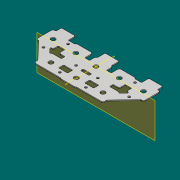
# Autodesk Inventor part: Part2
Saved by Autodesk Inventor 2018 (Build 220112000, 112)
## iProperties
Created: 2021-10-17
Part Number: Part2
Material: アルミニウム 6061
Document SubType Name: Modeling
Designer: gisen
Density: 2.7 g/cm^3
Appearance: アルミニウム - フラット
Author: gisen
Autodesk Inventor part; units mm, degrees
ref_plane "YZ Plane" through (0, 0, 0) normal (1, 0, 0) x (0, 1, 0)
ref_plane "XY Plane" through (0, 0, 0) normal (0, 0, 1) x (1, 0, 0)
ref_plane "作業平面1" through (0, -39.175, 8.3) normal (0, 0, -1) x (-1, 0, 0)
sketch "スケッチ1" plane through (0, -39.175, 8.3) normal (0, 0, -1) x (-1, 0, 0)
  arc A0 (-5.35, 6.375) -> (-6.35, 5.375) centre (-5.35, 5.375) ccw construction
  arc A1 (6.35, 5.375) -> (5.35, 6.375) centre (5.35, 5.375) ccw construction
  arc A2 (-32.9, 5.375) -> (-33.9, 6.375) centre (-33.9, 5.375) ccw construction
  arc A3 (-44.6, 6.375) -> (-45.6, 5.375) centre (-44.6, 5.375) ccw construction
  arc A4 (33.9, 6.375) -> (32.9, 5.375) centre (33.9, 5.375) ccw construction
  arc A5 (45.6, 5.375) -> (44.6, 6.375) centre (44.6, 5.375) ccw construction
  arc A6 (48.3, -0.325) -> (46.5, 1.475) centre (46.5, -0.325) ccw construction
  arc A7 (46.5, -13.925) -> (48.3, -12.125) centre (46.5, -12.125) ccw construction
  arc A8 (-46.5, 1.475) -> (-48.3, -0.325) centre (-46.5, -0.325) ccw construction
  arc A9 (-48.3, -12.125) -> (-46.5, -13.925) centre (-46.5, -12.125) ccw construction
  arc A10 (-17.5, -33.025) -> (-15.7, -31.225) centre (-17.5, -31.225) ccw construction
  arc A11 (15.7, -31.225) -> (17.5, -33.025) centre (17.5, -31.225) ccw construction
  arc A12 (31.1, -19.425) -> (29.3, -17.625) centre (29.3, -19.425) ccw construction
  arc A13 (-5.9, -0.585) -> (-7.7, -2.385) centre (-5.9, -2.385) ccw construction
  arc A14 (7.7, -2.385) -> (5.9, -0.585) centre (5.9, -2.385) ccw construction
  arc A15 (13.6, 0.875) -> (12.2994, 0.3193) centre (13.6, -0.925) ccw construction
  arc A16 (27.2, -0.925) -> (25.4, 0.875) centre (25.4, -0.925) ccw construction
  arc A17 (34.7, 1.475) -> (32.9, -0.325) centre (34.7, -0.325) ccw construction
  arc A18 (-12.2994, 0.3193) -> (-13.6, 0.875) centre (-13.6, -0.925) ccw construction
  arc A19 (-25.4, 0.875) -> (-27.2, -0.925) centre (-25.4, -0.925) ccw construction
  arc A20 (-32.9, -0.325) -> (-34.7, 1.475) centre (-34.7, -0.325) ccw construction
  arc A21 (-13.6, -14.525) -> (-11.8, -12.725) centre (-13.6, -12.725) ccw construction
  arc A22 (-3.25, -15.985) -> (-3.75, -16.485) centre (-3.25, -16.485) ccw construction
  arc A23 (-3.75, -17.725) -> (-3.25, -18.225) centre (-3.25, -17.725) ccw construction
  arc A24 (3.75, -16.485) -> (3.25, -15.985) centre (3.25, -16.485) ccw construction
  arc A25 (3.25, -18.225) -> (3.75, -17.725) centre (3.25, -17.725) ccw construction
  arc A26 (-15.7, -25.525) -> (-15.2, -26.025) centre (-15.2, -25.525) ccw construction
  arc A27 (-8.2, -26.025) -> (-7.7, -25.525) centre (-8.2, -25.525) ccw construction
  arc A28 (-15.2, -21.625) -> (-15.7, -22.125) centre (-15.2, -22.125) ccw construction
  arc A29 (-7.7, -22.125) -> (-8.2, -21.625) centre (-8.2, -22.125) ccw construction
  arc A30 (-7.317, -32.935) -> (-5.9, -33.625) centre (-5.9, -31.825) ccw construction
  arc A31 (5.9, -33.625) -> (7.317, -32.935) centre (5.9, -31.825) ccw construction
  line L0 (-7.4492, -33.025) -> (-17.5, -33.025) construction
  line L1 (17.5, -33.025) -> (7.4492, -33.025) construction
  line L2 (-31.306, -29.2915) -> (-45.7404, -14.0808) construction
  line L3 (45.7404, -14.0808) -> (31.306, -29.2915) construction
  arc A32 (-46.1, 1.475) -> (-45.6, 1.975) centre (-46.1, 1.975) ccw construction
  line L4 (-46.5, 1.375) -> (-46.1, 1.375)
  line L5 (-45.5, 1.975) -> (-45.5, 5.375)
  line L6 (-44.6, 6.275) -> (-33.9, 6.275)
  line L7 (-33, 5.375) -> (-33, 0.275)
  line L8 (-32.4, -0.325) -> (-27.3621, -0.325)
  arc A33 (-27.3621, -0.325) -> (-26.8503, -0.038) centre (-27.3621, 0.275) ccw
  arc A34 (-25.4, 0.775) -> (-26.8503, -0.038) centre (-25.4, -0.925) ccw
  line L9 (-25.4, 0.775) -> (-13.6, 0.775)
  line L10 (-11.9, -0.925) -> (-11.9, -5.875)
  line L11 (-11.3, -6.475) -> (-8.2, -6.475)
  line L12 (-7.6, -5.875) -> (-7.6, -2.385)
  arc A35 (-6.8321, -0.8452) -> (-6.35, 0.0103) centre (-7.35, 0.0103) ccw construction
  arc A36 (-6.7804, -0.9307) -> (-7.6, -2.385) centre (-5.9, -2.385) ccw
  arc A37 (-6.7804, -0.9307) -> (-6.25, 0.0103) centre (-7.35, 0.0103) ccw
  line L13 (-6.25, 0.0103) -> (-6.25, 5.375)
  line L14 (-5.35, 6.275) -> (5.35, 6.275)
  arc A38 (-5.35, 6.275) -> (-6.25, 5.375) centre (-5.35, 5.375) ccw
  arc A39 (-33, 5.375) -> (-33.9, 6.275) centre (-33.9, 5.375) ccw
  arc A40 (-44.6, 6.275) -> (-45.5, 5.375) centre (-44.6, 5.375) ccw
  arc A41 (-46.1, 1.375) -> (-45.5, 1.975) centre (-46.1, 1.975) ccw
  arc A42 (-33, 0.275) -> (-32.4, -0.325) centre (-32.4, 0.275) ccw
  arc A43 (-11.9, -5.875) -> (-11.3, -6.475) centre (-11.3, -5.875) ccw
  arc A44 (-8.2, -6.475) -> (-7.6, -5.875) centre (-8.2, -5.875) ccw
  arc A45 (-11.8, -5.875) -> (-11.3, -6.375) centre (-11.3, -5.875) ccw construction
  arc A46 (-8.2, -6.375) -> (-7.7, -5.875) centre (-8.2, -5.875) ccw construction
  arc A47 (-11.9, -0.925) -> (-13.6, 0.775) centre (-13.6, -0.925) ccw
  arc A48 (-32.9, 0.275) -> (-32.4, -0.225) centre (-32.4, 0.275) ccw construction
  arc A49 (-27.3621, -0.225) -> (-26.9356, 0.0141) centre (-27.3621, 0.275) ccw construction
  line L15 (-48.2, -0.325) -> (-48.2, -12.125)
  arc A50 (-48.2, -12.125) -> (-46.5, -13.825) centre (-46.5, -12.125) ccw
  line L16 (-45.6678, -14.012) -> (-31, -29.4687)
  arc A51 (-46.5, 1.375) -> (-48.2, -0.325) centre (-46.5, -0.325) ccw
  arc A52 (-45.7404, -14.0808) -> (-46.1031, -13.925) centre (-46.1031, -14.425) ccw construction
  line L17 (-17.5, -33.025) -> (-29.25, -33.025) construction
  line L18 (-31, -29.4687) -> (-31, -31.6478)
  line L19 (-31, -31.6478) -> (-29.788, -32.925)
  line L20 (-32.394, -30.324) -> (-30.1373, -32.7021) construction
  line L21 (-3.25, -15.985) -> (3.25, -15.985) construction
  line L22 (3.25, -18.225) -> (-3.25, -18.225) construction
  line L23 (0, -15.985) -> (0, -18.225) construction
  line L24 (-46.5, -13.925) -> (-46.1031, -13.925) construction
  line L25 (-15.2, -21.525) -> (-8.2, -21.525)
  line L26 (-7.6, -22.125) -> (-7.6, -25.525)
  line L27 (-8.2, -26.125) -> (-15.2, -26.125)
  line L28 (-15.8, -25.525) -> (-15.8, -22.125)
  line L29 (-3.25, -15.885) -> (3.25, -15.885)
  line L30 (3.85, -16.485) -> (3.85, -17.725)
  line L31 (3.25, -18.325) -> (-3.25, -18.325)
  line L32 (-3.85, -17.725) -> (-3.85, -16.485)
  arc A53 (-15.2, -21.525) -> (-15.8, -22.125) centre (-15.2, -22.125) ccw
  arc A54 (-7.6, -22.125) -> (-8.2, -21.525) centre (-8.2, -22.125) ccw
  arc A55 (-8.2, -26.125) -> (-7.6, -25.525) centre (-8.2, -25.525) ccw
  arc A56 (-15.8, -25.525) -> (-15.2, -26.125) centre (-15.2, -25.525) ccw
  arc A57 (-3.85, -17.725) -> (-3.25, -18.325) centre (-3.25, -17.725) ccw
  arc A58 (-3.25, -15.885) -> (-3.85, -16.485) centre (-3.25, -16.485) ccw
  arc A59 (3.85, -16.485) -> (3.25, -15.885) centre (3.25, -16.485) ccw
  arc A60 (3.25, -18.325) -> (3.85, -17.725) centre (3.25, -17.725) ccw
  line L33 (-29.788, -32.925) -> (-7.1961, -32.925)
  arc A61 (-7.1961, -32.925) -> (-5.9, -33.525) centre (-5.9, -31.825) ccw
  line L34 (-5.9, -33.525) -> (5.9, -33.525)
  line L35 (-5.9, -33.625) -> (5.9, -33.625) construction
  line L36 (-46.5, -13.825) -> (-46.1031, -13.825)
  arc A62 (-45.6678, -14.012) -> (-46.1031, -13.825) centre (-46.1031, -14.425) ccw
  line L37 (46.5, 1.375) -> (46.1, 1.375)
  line L38 (45.5, 1.975) -> (45.5, 5.375)
  line L39 (44.6, 6.275) -> (33.9, 6.275)
  line L40 (33, 5.375) -> (33, 0.275)
  line L41 (32.4, -0.325) -> (27.3621, -0.325)
  arc A63 (26.8503, -0.038) -> (27.3621, -0.325) centre (27.3621, 0.275) ccw
  arc A64 (26.8503, -0.038) -> (25.4, 0.775) centre (25.4, -0.925) ccw
  line L42 (25.4, 0.775) -> (13.6, 0.775)
  line L43 (11.9, -0.925) -> (11.9, -5.875)
  line L44 (11.3, -6.475) -> (8.2, -6.475)
  line L45 (7.6, -5.875) -> (7.6, -2.385)
  arc A65 (7.6, -2.385) -> (6.7804, -0.9307) centre (5.9, -2.385) ccw
  arc A66 (6.25, 0.0103) -> (6.7804, -0.9307) centre (7.35, 0.0103) ccw
  line L46 (6.25, 0.0103) -> (6.25, 5.375)
  arc A67 (6.25, 5.375) -> (5.35, 6.275) centre (5.35, 5.375) ccw
  arc A68 (33.9, 6.275) -> (33, 5.375) centre (33.9, 5.375) ccw
  arc A69 (45.5, 5.375) -> (44.6, 6.275) centre (44.6, 5.375) ccw
  arc A70 (45.5, 1.975) -> (46.1, 1.375) centre (46.1, 1.975) ccw
  arc A71 (32.4, -0.325) -> (33, 0.275) centre (32.4, 0.275) ccw
  arc A72 (11.3, -6.475) -> (11.9, -5.875) centre (11.3, -5.875) ccw
  arc A73 (7.6, -5.875) -> (8.2, -6.475) centre (8.2, -5.875) ccw
  arc A74 (13.6, 0.775) -> (11.9, -0.925) centre (13.6, -0.925) ccw
  line L47 (48.2, -0.325) -> (48.2, -12.125)
  arc A75 (46.5, -13.825) -> (48.2, -12.125) centre (46.5, -12.125) ccw
  line L48 (45.6678, -14.012) -> (31, -29.4687)
  arc A76 (48.2, -0.325) -> (46.5, 1.375) centre (46.5, -0.325) ccw
  line L49 (31, -29.4687) -> (31, -31.6478)
  line L50 (31, -31.6478) -> (29.788, -32.925)
  line L51 (15.2, -21.525) -> (8.2, -21.525)
  line L52 (7.6, -22.125) -> (7.6, -25.525)
  line L53 (8.2, -26.125) -> (15.2, -26.125)
  line L54 (15.8, -25.525) -> (15.8, -22.125)
  arc A77 (15.8, -22.125) -> (15.2, -21.525) centre (15.2, -22.125) ccw
  arc A78 (8.2, -21.525) -> (7.6, -22.125) centre (8.2, -22.125) ccw
  arc A79 (7.6, -25.525) -> (8.2, -26.125) centre (8.2, -25.525) ccw
  arc A80 (15.2, -26.125) -> (15.8, -25.525) centre (15.2, -25.525) ccw
  line L55 (29.788, -32.925) -> (7.1961, -32.925)
  arc A81 (5.9, -33.525) -> (7.1961, -32.925) centre (5.9, -31.825) ccw
  line L56 (46.5, -13.825) -> (46.1031, -13.825)
  arc A82 (46.1031, -13.825) -> (45.6678, -14.012) centre (46.1031, -14.425) ccw
  circle A83 centre (-38.492, -16.925) radius 0.8 construction
  circle A84 centre (-11.7, -29.025) radius 0.8 construction
  circle A85 centre (-9.75, -16.375) radius 0.8 construction
  circle A86 centre (-30.05, -3.225) radius 0.8 construction
  circle A87 centre (9.75, -16.375) radius 0.8 construction
  circle A88 centre (11.7, -29.025) radius 0.8 construction
  circle A89 centre (38.492, -16.925) radius 0.8 construction
  circle A90 centre (30.05, -3.225) radius 0.8 construction
  circle A91 centre (-30.05, -3.225) radius 1.05
  circle A92 centre (-38.492, -16.925) radius 1.05
  circle A93 centre (-11.7, -29.025) radius 1.05
  circle A94 centre (-9.75, -16.375) radius 1.05
  circle A95 centre (9.75, -16.375) radius 1.05
  circle A96 centre (11.7, -29.025) radius 1.05
  circle A97 centre (38.492, -16.925) radius 1.05
  circle A98 centre (30.05, -3.225) radius 1.05
  arc A99 (-32.394, -30.324) -> (-31.306, -29.2915) centre (-31.85, -29.8078) ccw projected
  line L57 (-45.7404, -14.0808) -> (-31.306, -29.2915) projected
  arc A100 (-45.7404, -14.0808) -> (-46.1031, -13.925) centre (-46.1031, -14.425) ccw projected
  arc A101 (-48.3, -12.125) -> (-46.5, -13.925) centre (-46.5, -12.125) ccw projected
  line L58 (-48.3, -0.539) -> (-48.3, -12.125) projected
  line L59 (-49, -0.539) -> (-48.3, -0.539) projected
  line L60 (-49, -12.426) -> (-49, -0.539) projected
  arc A102 (-49, -12.426) -> (-48.7254, -13.1144) centre (-48, -12.426) ccw projected
  line L61 (-32.394, -30.324) -> (-48.7254, -13.1144) projected
  arc A103 (-34.4677, -13.91) -> (-34.7659, -14.7499) centre (-34.4032, -14.4058) ccw construction
  line L62 (-34.7659, -14.7499) -> (-31.4157, -18.2803) construction
  arc A104 (-31.4157, -18.2803) -> (-30.672, -18.2598) centre (-31.0531, -17.9361) ccw construction
  arc A105 (-29.3, -17.625) -> (-30.672, -18.2598) centre (-29.3, -19.425) ccw construction
  line L63 (-22.2, -17.625) -> (-29.3, -17.625) construction
  arc A106 (-22.2, -17.625) -> (-21.7, -17.125) centre (-22.2, -17.125) ccw construction
  line L64 (-21.7, -15.025) -> (-21.7, -17.125) construction
  arc A107 (-21.7, -15.025) -> (-22.2, -14.525) centre (-22.2, -15.025) ccw construction
  line L65 (-25.4, -14.525) -> (-22.2, -14.525) construction
  arc A108 (-27.2, -12.725) -> (-25.4, -14.525) centre (-25.4, -12.725) ccw construction
  line L66 (-27.2, -9.725) -> (-27.2, -12.725) construction
  arc A109 (-27.2, -9.725) -> (-27.7, -9.225) centre (-27.7, -9.725) ccw construction
  line L67 (-32.4, -9.225) -> (-27.7, -9.225) construction
  arc A110 (-32.4, -9.225) -> (-32.9, -9.725) centre (-32.4, -9.725) ccw construction
  line L68 (-32.9, -12.125) -> (-32.9, -9.725) construction
  arc A111 (-34.4677, -13.91) -> (-32.9, -12.125) centre (-34.7, -12.125) ccw construction
  arc A112 (-27.1, -9.725) -> (-27.7, -9.125) centre (-27.7, -9.725) ccw
  line L69 (-27.1, -9.725) -> (-27.1, -12.725)
  arc A113 (-27.1, -12.725) -> (-25.4, -14.425) centre (-25.4, -12.725) ccw
  line L70 (-25.4, -14.425) -> (-22.2, -14.425)
  arc A114 (-21.6, -15.025) -> (-22.2, -14.425) centre (-22.2, -15.025) ccw
  line L71 (-21.6, -15.025) -> (-21.6, -17.125)
  arc A115 (-22.2, -17.725) -> (-21.6, -17.125) centre (-22.2, -17.125) ccw
  line L72 (-22.2, -17.725) -> (-29.3, -17.725)
  arc A116 (-29.3, -17.725) -> (-30.5957, -18.3245) centre (-29.3, -19.425) ccw
  arc A117 (-31.4883, -18.3491) -> (-30.5957, -18.3245) centre (-31.0531, -17.9361) ccw
  line L73 (-31.4883, -18.3491) -> (-34.8384, -14.8188)
  arc A118 (-34.4806, -13.8108) -> (-34.8384, -14.8188) centre (-34.4032, -14.4058) ccw
  arc A119 (-34.4806, -13.8108) -> (-33, -12.125) centre (-34.7, -12.125) ccw
  line L74 (-33, -12.125) -> (-33, -9.725)
  arc A120 (-32.4, -9.125) -> (-33, -9.725) centre (-32.4, -9.725) ccw
  line L75 (-32.4, -9.125) -> (-27.7, -9.125)
  arc A121 (30.672, -18.2598) -> (31.4157, -18.2803) centre (31.0531, -17.9361) ccw construction
  line L76 (31.4157, -18.2803) -> (34.7659, -14.7499) construction
  arc A122 (34.7659, -14.7499) -> (34.4677, -13.91) centre (34.4032, -14.4058) ccw construction
  arc A123 (32.9, -12.125) -> (34.4677, -13.91) centre (34.7, -12.125) ccw construction
  line L77 (32.9, -9.725) -> (32.9, -12.125) construction
  arc A124 (32.9, -9.725) -> (32.4, -9.225) centre (32.4, -9.725) ccw construction
  line L78 (27.7, -9.225) -> (32.4, -9.225) construction
  arc A125 (27.7, -9.225) -> (27.2, -9.725) centre (27.7, -9.725) ccw construction
  line L79 (27.2, -12.725) -> (27.2, -9.725) construction
  arc A126 (25.4, -14.525) -> (27.2, -12.725) centre (25.4, -12.725) ccw construction
  line L80 (22.2, -14.525) -> (25.4, -14.525) construction
  arc A127 (22.2, -14.525) -> (21.7, -15.025) centre (22.2, -15.025) ccw construction
  line L81 (21.7, -17.125) -> (21.7, -15.025) construction
  arc A128 (21.7, -17.125) -> (22.2, -17.625) centre (22.2, -17.125) ccw construction
  line L82 (29.3, -17.625) -> (22.2, -17.625) construction
  arc A129 (30.672, -18.2598) -> (29.3, -17.625) centre (29.3, -19.425) ccw construction
  arc A130 (27.7, -9.125) -> (27.1, -9.725) centre (27.7, -9.725) ccw
  line L83 (27.7, -9.125) -> (32.4, -9.125)
  arc A131 (33, -9.725) -> (32.4, -9.125) centre (32.4, -9.725) ccw
  line L84 (33, -9.725) -> (33, -12.125)
  arc A132 (33, -12.125) -> (34.4806, -13.8108) centre (34.7, -12.125) ccw
  arc A133 (34.8384, -14.8188) -> (34.4806, -13.8108) centre (34.4032, -14.4058) ccw
  line L85 (34.8384, -14.8188) -> (31.4883, -18.3491)
  arc A134 (30.5957, -18.3245) -> (31.4883, -18.3491) centre (31.0531, -17.9361) ccw
  arc A135 (30.5957, -18.3245) -> (29.3, -17.725) centre (29.3, -19.425) ccw
  line L86 (29.3, -17.725) -> (22.2, -17.725)
  arc A136 (21.6, -17.125) -> (22.2, -17.725) centre (22.2, -17.125) ccw
  line L87 (21.6, -17.125) -> (21.6, -15.025)
  arc A137 (22.2, -14.425) -> (21.6, -15.025) centre (22.2, -15.025) ccw
  line L88 (22.2, -14.425) -> (25.4, -14.425)
  arc A138 (25.4, -14.425) -> (27.1, -12.725) centre (25.4, -12.725) ccw
  line L89 (27.1, -12.725) -> (27.1, -9.725)
  point P0 (0, 39.175)
  point P1 (-34.992, -17.4172)
  point P2 (-31.7581, -20.825)
  point P3 (-31.6, -20.825)
  point P4 (-34.992, -14.425)
  point P5 (-31.1, -29.8078)
  dimension "d1" = 0.1
  dimension "d9" = 0.1
  dimension "d10" = 0.1
  dimension "d13" = 0.1
  dimension "d14" = 0.1
  dimension "d15" = 2.1
  dimension "d18" = 0.1
  dimension "d22" = 0.1
  dimension "d23" = 0.1
  constraints: 126 end point, 124 point on circle, 70 centre point, 61 symmetric about line, 45 tangent, 29 coincident, 19 equal radius, 9 perpendicular, 8 horizontal, 7 parallel, 4 vertical, 2 midpoint, 53 other
  measures "d1" distance from line of A0.start L14
  measures "d9" distance from line of L17 L19.end
  measures "d10" distance from line of L20 L18.end
  measures "d13" distance from line of A28.start L25
  measures "d14" distance between parallel lines of L34 L35
  measures "d15" diameter of A91
  measures "d18" distance from line of point (-31.1, -29.808) L18
  measures "d22" distance between parallel lines of L67 L75
  measures "d23" distance between parallel lines of L79 L89
extrude "押し出し1" add sketch "スケッチ1" along normal blind 0.8
sketch "スケッチ2" plane through (0, -39.175, 7.5) normal (0, 0, -1) x (-1, 0, 0)
  arc A0 (-46.5, 1.375) -> (-48.2, -0.325) centre (-46.5, -0.325) ccw construction
  arc A1 (-34.7, -13.825) -> (-33, -12.125) centre (-34.7, -12.125) ccw construction
  arc A2 (-25.4, 0.875) -> (-27.2, -0.925) centre (-25.4, -0.925) ccw construction
  arc A3 (-13.6, -14.525) -> (-11.8, -12.725) centre (-13.6, -12.725) ccw construction
  arc A4 (-5.9, -0.585) -> (-7.7, -2.385) centre (-5.9, -2.385) ccw construction
  arc A5 (5.9, -15.985) -> (7.7, -14.185) centre (5.9, -14.185) ccw construction
  arc A6 (-29.3, -17.625) -> (-31.1, -19.425) centre (-29.3, -19.425) ccw construction
  arc A7 (-17.5, -33.025) -> (-15.7, -31.225) centre (-17.5, -31.225) ccw construction
  arc A8 (-5.9, -18.225) -> (-7.7, -20.025) centre (-5.9, -20.025) ccw construction
  arc A9 (7.317, -32.935) -> (7.7, -31.825) centre (5.9, -31.825) ccw construction
  arc A10 (15.7, -31.225) -> (17.5, -33.025) centre (17.5, -31.225) ccw construction
  arc A11 (31.1, -19.425) -> (29.3, -17.625) centre (29.3, -19.425) ccw construction
  arc A12 (11.8, -12.725) -> (13.6, -14.525) centre (13.6, -12.725) ccw construction
  arc A13 (27.2, -0.925) -> (25.4, 0.875) centre (25.4, -0.925) ccw construction
  arc A14 (32.9, -12.125) -> (34.7, -13.925) centre (34.7, -12.125) ccw construction
  arc A15 (48.3, -0.325) -> (46.5, 1.475) centre (46.5, -0.325) ccw construction
  line L0 (-46.5, -0.325) -> (-34.7, -12.125) construction
  line L1 (-25.4, -0.925) -> (-13.6, -12.725) construction
  line L2 (-5.9, -2.385) -> (5.9, -14.185) construction
  line L3 (13.6, -12.725) -> (25.4, -0.925) construction
  line L4 (34.7, -12.125) -> (46.5, -0.325) construction
  line L5 (29.3, -19.425) -> (17.5, -31.225) construction
  line L6 (-5.9, -20.025) -> (5.9, -31.825) construction
  line L7 (-29.3, -19.425) -> (-17.5, -31.225) construction
  circle A16 centre (-40.6, -6.225) radius 2
  circle A17 centre (-19.5, -6.825) radius 2
  circle A18 centre (0, -8.285) radius 2
  circle A19 centre (19.5, -6.825) radius 2
  circle A20 centre (40.6, -6.225) radius 2
  circle A21 centre (23.4, -25.325) radius 2
  circle A22 centre (0, -25.925) radius 2
  circle A23 centre (-23.4, -25.325) radius 2
  point P0 (0, 39.175)
  dimension "d19" = 4
  constraints: 16 end point, 8 centre point, 8 midpoint, 7 equal radius
  measures "d19" diameter of A16
extrude "押し出し2" cut sketch "スケッチ2" against normal through all
ref_plane "作業平面3" through (0, -51.3, 8.3) normal (-1, 0, 0) x (0, 0, 1)
ref_plane "作業平面4" through (0, -47.46, 0) normal (0, 1, 0) x (-1, 0, 0)
equation "\"d9\" = d1"
equation "\"d10\" = d1"
equation "\"d13\" = d1"
equation "\"d14\" = d1"
equation "\"d18\" = d1"
